Autodesk Fusion 360 part; units mm, degrees
(part 2 of 2)
sketch "Sketch2 (3)" plane through (0, 0, -6.4) normal (0, 0, -1) x (1, 0, 0) in component "Holding Plate"
  arc A0 (121.6882, 36.141) -> (112.1882, 45.641) centre (112.1882, 36.141) ccw
  line L0 (112.1882, 45.641) -> (14.8614, 45.641)
  line L1 (14.8614, 45.641) -> (14.8614, -58.688)
  line L2 (14.8614, -58.688) -> (98.2844, -58.688)
  line L3 (98.2844, -58.688) -> (98.2844, -66.2117)
  line L4 (98.2844, -66.2117) -> (121.1297, -66.2117)
  line L5 (121.1297, -66.2117) -> (121.1297, -42.1871)
  line L6 (121.1297, -42.1871) -> (101.4385, -42.1871)
  line L7 (101.4385, -42.1871) -> (101.4385, 27.1211)
  line L8 (101.4385, 27.1211) -> (121.6882, 27.1211)
  line L9 (121.6882, 27.1211) -> (121.6882, 36.141)
  line L10 (20, -40) -> (27.5, -40)
  line L11 (27.5, -40) -> (27.5, -43)
  line L12 (27.5, -43) -> (30.5, -43)
  line L13 (30.5, -43) -> (30.5, -49.2)
  line L14 (30.5, -49.2) -> (25.4, -49.2)
  line L15 (25.4, -49.2) -> (25.4, -54.4)
  line L16 (25.4, -54.4) -> (20, -54.4)
  line L17 (20, -54.4) -> (20, -40)
  line L18 (73.4, -1.6) -> (73.4, 0)
  line L19 (73.4, 0) -> (75, 0)
  line L20 (75, 0) -> (75, -1.6)
  line L21 (75, -1.6) -> (73.4, -1.6)
  line L22 (60, -40) -> (67.5, -40)
  line L23 (67.5, -40) -> (67.5, -43)
  line L24 (67.5, -43) -> (70.5, -43)
  line L25 (70.5, -43) -> (70.5, -49.2)
  line L26 (70.5, -49.2) -> (65.4, -49.2)
  line L27 (65.4, -49.2) -> (65.4, -54.4)
  line L28 (65.4, -54.4) -> (60, -54.4)
  line L29 (60, -54.4) -> (60, -40)
  line L30 (33.4, -41.6) -> (33.4, -40)
  line L31 (33.4, -40) -> (35, -40)
  line L32 (35, -40) -> (35, -41.6)
  line L33 (35, -41.6) -> (33.4, -41.6)
  line L34 (80, 20) -> (87.5, 20)
  line L35 (87.5, 20) -> (87.5, 17)
  line L36 (87.5, 17) -> (90.5, 17)
  line L37 (90.5, 17) -> (90.5, 10.8)
  line L38 (90.5, 10.8) -> (85.4, 10.8)
  line L39 (85.4, 10.8) -> (85.4, 5.6)
  line L40 (85.4, 5.6) -> (80, 5.6)
  line L41 (80, 5.6) -> (80, 20)
  line L42 (53.4, -41.6) -> (53.4, -40)
  line L43 (53.4, -40) -> (55, -40)
  line L44 (55, -40) -> (55, -41.6)
  line L45 (55, -41.6) -> (53.4, -41.6)
  line L46 (93.4, -1.6) -> (93.4, 0)
  line L47 (93.4, 0) -> (95, 0)
  line L48 (95, 0) -> (95, -1.6)
  line L49 (95, -1.6) -> (93.4, -1.6)
  line L50 (75, -52.8) -> (75, -54.4)
  line L51 (75, -54.4) -> (73.4, -54.4)
  line L52 (73.4, -54.4) -> (73.4, -52.8)
  line L53 (73.4, -52.8) -> (75, -52.8)
  line L54 (40, -40) -> (47.5, -40)
  line L55 (47.5, -40) -> (47.5, -43)
  line L56 (47.5, -43) -> (50.5, -43)
  line L57 (50.5, -43) -> (50.5, -49.2)
  line L58 (50.5, -49.2) -> (45.4, -49.2)
  line L59 (45.4, -49.2) -> (45.4, -54.4)
  line L60 (45.4, -54.4) -> (40, -54.4)
  line L61 (40, -54.4) -> (40, -40)
  line L62 (55, -52.8) -> (55, -54.4)
  line L63 (55, -54.4) -> (53.4, -54.4)
  line L64 (53.4, -54.4) -> (53.4, -52.8)
  line L65 (53.4, -52.8) -> (55, -52.8)
  line L66 (80, -20) -> (87.5, -20)
  line L67 (87.5, -20) -> (87.5, -23)
  line L68 (87.5, -23) -> (90.5, -23)
  line L69 (90.5, -23) -> (90.5, -29.2)
  line L70 (90.5, -29.2) -> (85.4, -29.2)
  line L71 (85.4, -29.2) -> (85.4, -34.4)
  line L72 (85.4, -34.4) -> (80, -34.4)
  line L73 (80, -34.4) -> (80, -20)
  line L74 (60, -20) -> (67.5, -20)
  line L75 (67.5, -20) -> (67.5, -23)
  line L76 (67.5, -23) -> (70.5, -23)
  line L77 (70.5, -23) -> (70.5, -29.2)
  line L78 (70.5, -29.2) -> (65.4, -29.2)
  line L79 (65.4, -29.2) -> (65.4, -34.4)
  line L80 (65.4, -34.4) -> (60, -34.4)
  line L81 (60, -34.4) -> (60, -20)
  line L82 (93.4, -21.6) -> (93.4, -20)
  line L83 (93.4, -20) -> (95, -20)
  line L84 (95, -20) -> (95, -21.6)
  line L85 (95, -21.6) -> (93.4, -21.6)
  line L86 (80, -40) -> (87.5, -40)
  line L87 (87.5, -40) -> (87.5, -43)
  line L88 (87.5, -43) -> (90.5, -43)
  line L89 (90.5, -43) -> (90.5, -49.2)
  line L90 (90.5, -49.2) -> (85.4, -49.2)
  line L91 (85.4, -49.2) -> (85.4, -54.4)
  line L92 (85.4, -54.4) -> (80, -54.4)
  line L93 (80, -54.4) -> (80, -40)
  line L94 (95, -54.4) -> (93.4, -54.4)
  line L95 (93.4, -54.4) -> (93.4, -52.8)
  line L96 (93.4, -52.8) -> (95, -52.8)
  line L97 (95, -52.8) -> (95, -54.4)
  line L98 (35, -52.8) -> (35, -54.4)
  line L99 (35, -54.4) -> (33.4, -54.4)
  line L100 (33.4, -54.4) -> (33.4, -52.8)
  line L101 (33.4, -52.8) -> (35, -52.8)
  line L102 (95, -12.8) -> (95, -14.4)
  line L103 (95, -14.4) -> (93.4, -14.4)
  line L104 (93.4, -14.4) -> (93.4, -12.8)
  line L105 (93.4, -12.8) -> (95, -12.8)
  line L106 (60, 0) -> (67.5, 0)
  line L107 (67.5, 0) -> (67.5, -3)
  line L108 (67.5, -3) -> (70.5, -3)
  line L109 (70.5, -3) -> (70.5, -9.2)
  line L110 (70.5, -9.2) -> (65.4, -9.2)
  line L111 (65.4, -9.2) -> (65.4, -14.4)
  line L112 (65.4, -14.4) -> (60, -14.4)
  line L113 (60, -14.4) -> (60, 0)
  line L114 (75, 7.2) -> (75, 5.6)
  line L115 (75, 5.6) -> (73.4, 5.6)
  line L116 (73.4, 5.6) -> (73.4, 7.2)
  line L117 (73.4, 7.2) -> (75, 7.2)
  line L118 (73.4, -21.6) -> (73.4, -20)
  line L119 (73.4, -20) -> (75, -20)
  line L120 (75, -20) -> (75, -21.6)
  line L121 (75, -21.6) -> (73.4, -21.6)
  line L122 (73.4, -41.6) -> (73.4, -40)
  line L123 (73.4, -40) -> (75, -40)
  line L124 (75, -40) -> (75, -41.6)
  line L125 (75, -41.6) -> (73.4, -41.6)
  line L126 (95, -32.8) -> (95, -34.4)
  line L127 (95, -34.4) -> (93.4, -34.4)
  line L128 (93.4, -34.4) -> (93.4, -32.8)
  line L129 (93.4, -32.8) -> (95, -32.8)
  line L130 (75, -32.8) -> (75, -34.4)
  line L131 (75, -34.4) -> (73.4, -34.4)
  line L132 (73.4, -34.4) -> (73.4, -32.8)
  line L133 (73.4, -32.8) -> (75, -32.8)
  line L134 (93.4, 18.4) -> (93.4, 20)
  line L135 (93.4, 20) -> (95, 20)
  line L136 (95, 20) -> (95, 18.4)
  line L137 (95, 18.4) -> (93.4, 18.4)
  line L138 (95, 7.2) -> (95, 5.6)
  line L139 (95, 5.6) -> (93.4, 5.6)
  line L140 (93.4, 5.6) -> (93.4, 7.2)
  line L141 (93.4, 7.2) -> (95, 7.2)
  line L142 (93.4, -41.6) -> (93.4, -40)
  line L143 (93.4, -40) -> (95, -40)
  line L144 (95, -40) -> (95, -41.6)
  line L145 (95, -41.6) -> (93.4, -41.6)
  line L146 (75, -12.8) -> (75, -14.4)
  line L147 (75, -14.4) -> (73.4, -14.4)
  line L148 (73.4, -14.4) -> (73.4, -12.8)
  line L149 (73.4, -12.8) -> (75, -12.8)
  line L150 (80, 0) -> (87.5, 0)
  line L151 (87.5, 0) -> (87.5, -3)
  line L152 (87.5, -3) -> (90.5, -3)
  line L153 (90.5, -3) -> (90.5, -9.2)
  line L154 (90.5, -9.2) -> (85.4, -9.2)
  line L155 (85.4, -9.2) -> (85.4, -14.4)
  line L156 (85.4, -14.4) -> (80, -14.4)
  line L157 (80, -14.4) -> (80, 0)
  line L158 (73.4, 18.4) -> (73.4, 20)
  line L159 (73.4, 20) -> (75, 20)
  line L160 (75, 20) -> (75, 18.4)
  line L161 (75, 18.4) -> (73.4, 18.4)
  line L162 (60, 20) -> (67.5, 20)
  line L163 (67.5, 20) -> (67.5, 17)
  line L164 (67.5, 17) -> (70.5, 17)
  line L165 (70.5, 17) -> (70.5, 10.8)
  line L166 (70.5, 10.8) -> (65.4, 10.8)
  line L167 (65.4, 10.8) -> (65.4, 5.6)
  line L168 (65.4, 5.6) -> (60, 5.6)
  line L169 (60, 5.6) -> (60, 20)
  line L170 (40, 40) -> (47.5, 40)
  line L171 (47.5, 40) -> (47.5, 37)
  line L172 (47.5, 37) -> (50.5, 37)
  line L173 (50.5, 37) -> (50.5, 30.8)
  line L174 (50.5, 30.8) -> (45.4, 30.8)
  line L175 (45.4, 30.8) -> (45.4, 25.6)
  line L176 (45.4, 25.6) -> (40, 25.6)
  line L177 (40, 25.6) -> (40, 40)
  line L178 (55, 27.2) -> (55, 25.6)
  line L179 (55, 25.6) -> (53.4, 25.6)
  line L180 (53.4, 25.6) -> (53.4, 27.2)
  line L181 (53.4, 27.2) -> (55, 27.2)
  line L182 (60, 40) -> (67.5, 40)
  line L183 (67.5, 40) -> (67.5, 37)
  line L184 (67.5, 37) -> (70.5, 37)
  line L185 (70.5, 37) -> (70.5, 30.8)
  line L186 (70.5, 30.8) -> (65.4, 30.8)
  line L187 (65.4, 30.8) -> (65.4, 25.6)
  line L188 (65.4, 25.6) -> (60, 25.6)
  line L189 (60, 25.6) -> (60, 40)
  line L190 (80, 40) -> (87.5, 40)
  line L191 (87.5, 40) -> (87.5, 37)
  line L192 (87.5, 37) -> (90.5, 37)
  line L193 (90.5, 37) -> (90.5, 30.8)
  line L194 (90.5, 30.8) -> (85.4, 30.8)
  line L195 (85.4, 30.8) -> (85.4, 25.6)
  line L196 (85.4, 25.6) -> (80, 25.6)
  line L197 (80, 25.6) -> (80, 40)
  line L198 (93.4, 38.4) -> (93.4, 40)
  line L199 (93.4, 40) -> (95, 40)
  line L200 (95, 40) -> (95, 38.4)
  line L201 (95, 38.4) -> (93.4, 38.4)
  line L202 (95, 27.2) -> (95, 25.6)
  line L203 (95, 25.6) -> (93.4, 25.6)
  line L204 (93.4, 25.6) -> (93.4, 27.2)
  line L205 (93.4, 27.2) -> (95, 27.2)
  line L206 (53.4, 38.4) -> (53.4, 40)
  line L207 (53.4, 40) -> (55, 40)
  line L208 (55, 40) -> (55, 38.4)
  line L209 (55, 38.4) -> (53.4, 38.4)
  line L210 (75, 27.2) -> (75, 25.6)
  line L211 (75, 25.6) -> (73.4, 25.6)
  line L212 (73.4, 25.6) -> (73.4, 27.2)
  line L213 (73.4, 27.2) -> (75, 27.2)
  line L214 (73.4, 38.4) -> (73.4, 40)
  line L215 (73.4, 40) -> (75, 40)
  line L216 (75, 40) -> (75, 38.4)
  line L217 (75, 38.4) -> (73.4, 38.4)
  circle A1 centre (28.0569, 26.8711) radius 5
  circle A2 centre (36.7164, -15.9226) radius 5
  circle A3 centre (109.0489, 35.4607) radius 5
  circle A4 centre (109.0489, -55.2728) radius 5
  dimension "d163" = 10
  dimension "d164" = 10
  dimension "d189" = 10
  dimension "d190" = 10
  measures "d163" diameter of A1
  measures "d164" diameter of A2
  measures "d189" diameter of A3
  measures "d190" diameter of A4
extrude "Extrude2''" add sketch "Sketch2 (3)" along normal blind 14.5 contours A1 | A2 | A3 | A4 bodies 3 in component "Holding Plate"
sketch "Sketch3 (3)" plane through (0, 0, 0) normal (0, 0, -1) x (1, 0, 0)
  arc A0 (123.05, 36.8) -> (113.05, 46.8) centre (113.05, 36.8) ccw
  line L0 (113.05, 46.8) -> (-34, 46.8)
  arc A1 (-34, 46.8) -> (-44, 36.8) centre (-34, 36.8) ccw
  line L1 (-44, 36.8) -> (-44, -87.5)
  arc A2 (-44, -87.5) -> (-34, -97.5) centre (-34, -87.5) ccw
  line L2 (-34, -97.5) -> (27.575, -97.5)
  line L3 (27.575, -97.5) -> (27.575, -75.5)
  line L4 (27.575, -75.5) -> (30.425, -75.5)
  line L5 (30.425, -75.5) -> (30.425, -97.5)
  line L6 (48.625, -97.5) -> (48.625, -75.5)
  line L7 (48.625, -75.5) -> (51.475, -75.5)
  line L8 (51.475, -75.5) -> (51.475, -97.5)
  line L9 (51.475, -97.5) -> (113.05, -97.5)
  arc A3 (113.05, -97.5) -> (123.05, -87.5) centre (113.05, -87.5) ccw
  line L10 (123.05, -87.5) -> (123.05, 36.8)
  line L11 (59.4, -55.25) -> (59.4, -39.15)
  line L12 (59.4, -39.15) -> (75.6, -39.15)
  line L13 (75.6, -39.15) -> (75.6, -55.25)
  line L14 (75.6, -55.25) -> (59.4, -55.25)
  line L15 (59.4, -15.25) -> (59.4, 0.85)
  line L16 (59.4, 0.85) -> (75.6, 0.85)
  line L17 (75.6, 0.85) -> (75.6, -15.25)
  line L18 (75.6, -15.25) -> (59.4, -15.25)
  line L19 (39.4, 24.75) -> (39.4, 40.85)
  line L20 (39.4, 40.85) -> (55.6, 40.85)
  line L21 (55.6, 40.85) -> (55.6, 24.75)
  line L22 (55.6, 24.75) -> (39.4, 24.75)
  line L23 (59.4, 24.75) -> (59.4, 40.85)
  line L24 (59.4, 40.85) -> (75.6, 40.85)
  line L25 (75.6, 40.85) -> (75.6, 24.75)
  line L26 (75.6, 24.75) -> (59.4, 24.75)
  line L27 (79.4, -15.25) -> (79.4, 0.85)
  line L28 (79.4, 0.85) -> (95.6, 0.85)
  line L29 (95.6, 0.85) -> (95.6, -15.25)
  line L30 (95.6, -15.25) -> (79.4, -15.25)
  line L31 (79.4, -55.25) -> (79.4, -39.15)
  line L32 (79.4, -39.15) -> (95.6, -39.15)
  line L33 (95.6, -39.15) -> (95.6, -55.25)
  line L34 (95.6, -55.25) -> (79.4, -55.25)
  line L35 (39.4, -55.25) -> (39.4, -39.15)
  line L36 (39.4, -39.15) -> (55.6, -39.15)
  line L37 (55.6, -39.15) -> (55.6, -55.25)
  line L38 (55.6, -55.25) -> (39.4, -55.25)
  line L39 (79.4, -35.25) -> (79.4, -19.15)
  line L40 (79.4, -19.15) -> (95.6, -19.15)
  line L41 (95.6, -19.15) -> (95.6, -35.25)
  line L42 (95.6, -35.25) -> (79.4, -35.25)
  line L43 (59.4, 4.75) -> (59.4, 20.85)
  line L44 (59.4, 20.85) -> (75.6, 20.85)
  line L45 (75.6, 20.85) -> (75.6, 4.75)
  line L46 (75.6, 4.75) -> (59.4, 4.75)
  line L47 (79.4, 24.75) -> (79.4, 40.85)
  line L48 (79.4, 40.85) -> (95.6, 40.85)
  line L49 (95.6, 40.85) -> (95.6, 24.75)
  line L50 (95.6, 24.75) -> (79.4, 24.75)
  line L51 (79.4, 4.75) -> (79.4, 20.85)
  line L52 (79.4, 20.85) -> (95.6, 20.85)
  line L53 (95.6, 20.85) -> (95.6, 4.75)
  line L54 (95.6, 4.75) -> (79.4, 4.75)
  line L55 (59.4, -35.25) -> (59.4, -19.15)
  line L56 (59.4, -19.15) -> (75.6, -19.15)
  line L57 (75.6, -19.15) -> (75.6, -35.25)
  line L58 (75.6, -35.25) -> (59.4, -35.25)
  line L59 (19.4, -55.25) -> (19.4, -39.15)
  line L60 (19.4, -39.15) -> (35.6, -39.15)
  line L61 (35.6, -39.15) -> (35.6, -55.25)
  line L62 (35.6, -55.25) -> (19.4, -55.25)
  circle A4 centre (112, -33.75) radius 2.75
  circle A5 centre (112, 19.35) radius 2.75
  circle A6 centre (-20.7, -75) radius 3.675
  circle A7 centre (19.3, -75) radius 3.675
  circle A8 centre (59.3, -75) radius 3.675
  circle A9 centre (99.3, -75) radius 3.675
  circle A10 centre (112, -7.2) radius 6.25
  circle A11 centre (0, 0) radius 3.675
  circle A12 centre (-26.1553, -31.0832) radius 5
  circle A13 centre (80.0291, -77.7504) radius 5
  circle A14 centre (-20.8711, 13.9931) radius 5
  line L63 (30.425, -97.5) -> (48.625, -97.5)
  circle A15 centre (-1.1738, -82.7474) radius 5
  dimension "d167" = 10
  dimension "d170" = 10
  dimension "d171" = 10
  dimension "d176" = 10
  measures "d167" diameter of A12
  measures "d170" diameter of A13
  measures "d171" diameter of A14
  measures "d176" diameter of A15
extrude "Extrude14" add sketch "Sketch3 (3)" along normal blind 21 contours A12 | A13 | A14 | A15 bodies 1 in component "Top"
sketch "Sketch11" plane through (0, 0, 0) normal (0, 0, -1) x (1, 0, 0) in component "Top"
  circle A0 centre (-1.1738, -82.7474) radius 5
  circle A1 centre (-26.1553, -31.0832) radius 5
  circle A2 centre (80.0291, -77.7504) radius 5
  circle A3 centre (-20.8711, 13.9931) radius 5
  arc A4 (123.05, 36.8) -> (113.05, 46.8) centre (113.05, 36.8) ccw
  line L0 (113.05, 46.8) -> (-34, 46.8)
  arc A5 (-34, 46.8) -> (-44, 36.8) centre (-34, 36.8) ccw
  line L1 (-44, 36.8) -> (-44, -87.5)
  arc A6 (-44, -87.5) -> (-34, -97.5) centre (-34, -87.5) ccw
  line L2 (-34, -97.5) -> (27.575, -97.5)
  line L3 (27.575, -97.5) -> (27.575, -75.5)
  line L4 (27.575, -75.5) -> (30.425, -75.5)
  line L5 (30.425, -75.5) -> (30.425, -97.5)
  line L6 (30.425, -97.5) -> (48.625, -97.5)
  line L7 (48.625, -97.5) -> (48.625, -75.5)
  line L8 (48.625, -75.5) -> (51.475, -75.5)
  line L9 (51.475, -75.5) -> (51.475, -97.5)
  line L10 (51.475, -97.5) -> (113.05, -97.5)
  arc A7 (113.05, -97.5) -> (123.05, -87.5) centre (113.05, -87.5) ccw
  line L11 (123.05, -87.5) -> (123.05, 36.8)
  line L12 (59.4, -55.25) -> (59.4, -39.15)
  line L13 (59.4, -39.15) -> (75.6, -39.15)
  line L14 (75.6, -39.15) -> (75.6, -55.25)
  line L15 (75.6, -55.25) -> (59.4, -55.25)
  line L16 (59.4, -15.25) -> (59.4, 0.85)
  line L17 (59.4, 0.85) -> (75.6, 0.85)
  line L18 (75.6, 0.85) -> (75.6, -15.25)
  line L19 (75.6, -15.25) -> (59.4, -15.25)
  line L20 (39.4, 24.75) -> (39.4, 40.85)
  line L21 (39.4, 40.85) -> (55.6, 40.85)
  line L22 (55.6, 40.85) -> (55.6, 24.75)
  line L23 (55.6, 24.75) -> (39.4, 24.75)
  line L24 (59.4, 24.75) -> (59.4, 40.85)
  line L25 (59.4, 40.85) -> (75.6, 40.85)
  line L26 (75.6, 40.85) -> (75.6, 24.75)
  line L27 (75.6, 24.75) -> (59.4, 24.75)
  line L28 (79.4, -15.25) -> (79.4, 0.85)
  line L29 (79.4, 0.85) -> (95.6, 0.85)
  line L30 (95.6, 0.85) -> (95.6, -15.25)
  line L31 (95.6, -15.25) -> (79.4, -15.25)
  line L32 (79.4, -55.25) -> (79.4, -39.15)
  line L33 (79.4, -39.15) -> (95.6, -39.15)
  line L34 (95.6, -39.15) -> (95.6, -55.25)
  line L35 (95.6, -55.25) -> (79.4, -55.25)
  line L36 (39.4, -55.25) -> (39.4, -39.15)
  line L37 (39.4, -39.15) -> (55.6, -39.15)
  line L38 (55.6, -39.15) -> (55.6, -55.25)
  line L39 (55.6, -55.25) -> (39.4, -55.25)
  line L40 (79.4, -35.25) -> (79.4, -19.15)
  line L41 (79.4, -19.15) -> (95.6, -19.15)
  line L42 (95.6, -19.15) -> (95.6, -35.25)
  line L43 (95.6, -35.25) -> (79.4, -35.25)
  line L44 (59.4, 4.75) -> (59.4, 20.85)
  line L45 (59.4, 20.85) -> (75.6, 20.85)
  line L46 (75.6, 20.85) -> (75.6, 4.75)
  line L47 (75.6, 4.75) -> (59.4, 4.75)
  line L48 (79.4, 24.75) -> (79.4, 40.85)
  line L49 (79.4, 40.85) -> (95.6, 40.85)
  line L50 (95.6, 40.85) -> (95.6, 24.75)
  line L51 (95.6, 24.75) -> (79.4, 24.75)
  line L52 (79.4, 4.75) -> (79.4, 20.85)
  line L53 (79.4, 20.85) -> (95.6, 20.85)
  line L54 (95.6, 20.85) -> (95.6, 4.75)
  line L55 (95.6, 4.75) -> (79.4, 4.75)
  line L56 (59.4, -35.25) -> (59.4, -19.15)
  line L57 (59.4, -19.15) -> (75.6, -19.15)
  line L58 (75.6, -19.15) -> (75.6, -35.25)
  line L59 (75.6, -35.25) -> (59.4, -35.25)
  line L60 (19.4, -55.25) -> (19.4, -39.15)
  line L61 (19.4, -39.15) -> (35.6, -39.15)
  line L62 (35.6, -39.15) -> (35.6, -55.25)
  line L63 (35.6, -55.25) -> (19.4, -55.25)
  circle A8 centre (112, -33.75) radius 2.75
  circle A9 centre (112, 19.35) radius 2.75
  circle A10 centre (-20.7, -75) radius 3.675
  circle A11 centre (19.3, -75) radius 3.675
  circle A12 centre (59.3, -75) radius 3.675
  circle A13 centre (99.3, -75) radius 3.675
  circle A14 centre (112, -7.2) radius 6.25
  circle A15 centre (0, 0) radius 3.675
  circle A16 centre (35.815, -26.5694) radius 5
  circle A17 centre (34.6117, 12.124) radius 5
  circle A18 centre (109.9321, -52.4845) radius 5
  circle A19 centre (107.0903, 35.1385) radius 5
  dimension "d177" = 10
  dimension "d178" = 10
  dimension "d179" = 10
  dimension "d180" = 10
  measures "d177" diameter of A16
  measures "d178" diameter of A17
  measures "d179" diameter of A18
  measures "d180" diameter of A19
extrude "Extrude15" add sketch "Sketch11" along normal blind 5.2 contours A16 | A17 | A18 bodies 1 in component "Top"
sketch "Sketch3 (4)" plane through (0, 0, -4.4) normal (0, 0, 1) x (-1, 0, 0) in component "Holding Plate"
  arc A0 (-112.1882, 45.641) -> (-121.6882, 36.141) centre (-112.1882, 36.141) ccw
  line L0 (-121.6882, 36.141) -> (-121.6882, 27.1211)
  line L1 (-121.6882, 27.1211) -> (-101.4385, 27.1211)
  line L2 (-101.4385, 27.1211) -> (-101.4385, -42.1871)
  line L3 (-101.4385, -42.1871) -> (-121.1297, -42.1871)
  line L4 (-121.1297, -42.1871) -> (-121.1297, -66.2117)
  line L5 (-121.1297, -66.2117) -> (-98.2844, -66.2117)
  line L6 (-98.2844, -66.2117) -> (-98.2844, -58.688)
  line L7 (-98.2844, -58.688) -> (-14.8614, -58.688)
  line L8 (-14.8614, -58.688) -> (-14.8614, 45.641)
  line L9 (-14.8614, 45.641) -> (-112.1882, 45.641)
  line L10 (-93.4, -54.4) -> (-95, -54.4)
  line L11 (-95, -54.4) -> (-95, -52.8)
  line L12 (-95, -52.8) -> (-93.4, -52.8)
  line L13 (-93.4, -52.8) -> (-93.4, -54.4)
  line L14 (-93.4, -40) -> (-93.4, -41.6)
  line L15 (-93.4, -41.6) -> (-95, -41.6)
  line L16 (-95, -41.6) -> (-95, -40)
  line L17 (-95, -40) -> (-93.4, -40)
  line L18 (-73.4, -40) -> (-73.4, -41.6)
  line L19 (-73.4, -41.6) -> (-75, -41.6)
  line L20 (-75, -41.6) -> (-75, -40)
  line L21 (-75, -40) -> (-73.4, -40)
  line L22 (-87.5, -40) -> (-80, -40)
  line L23 (-80, -40) -> (-80, -54.4)
  line L24 (-80, -54.4) -> (-85.4, -54.4)
  line L25 (-85.4, -54.4) -> (-85.4, -49.2)
  line L26 (-85.4, -49.2) -> (-90.5, -49.2)
  line L27 (-90.5, -49.2) -> (-90.5, -43)
  line L28 (-90.5, -43) -> (-87.5, -43)
  line L29 (-87.5, -43) -> (-87.5, -40)
  line L30 (-75, -54.4) -> (-75, -52.8)
  line L31 (-75, -52.8) -> (-73.4, -52.8)
  line L32 (-73.4, -52.8) -> (-73.4, -54.4)
  line L33 (-73.4, -54.4) -> (-75, -54.4)
  line L34 (-47.5, -40) -> (-40, -40)
  line L35 (-40, -40) -> (-40, -54.4)
  line L36 (-40, -54.4) -> (-45.4, -54.4)
  line L37 (-45.4, -54.4) -> (-45.4, -49.2)
  line L38 (-45.4, -49.2) -> (-50.5, -49.2)
  line L39 (-50.5, -49.2) -> (-50.5, -43)
  line L40 (-50.5, -43) -> (-47.5, -43)
  line L41 (-47.5, -43) -> (-47.5, -40)
  line L42 (-87.5, 0) -> (-80, 0)
  line L43 (-80, 0) -> (-80, -14.4)
  line L44 (-80, -14.4) -> (-85.4, -14.4)
  line L45 (-85.4, -14.4) -> (-85.4, -9.2)
  line L46 (-85.4, -9.2) -> (-90.5, -9.2)
  line L47 (-90.5, -9.2) -> (-90.5, -3)
  line L48 (-90.5, -3) -> (-87.5, -3)
  line L49 (-87.5, -3) -> (-87.5, 0)
  line L50 (-87.5, -20) -> (-80, -20)
  line L51 (-80, -20) -> (-80, -34.4)
  line L52 (-80, -34.4) -> (-85.4, -34.4)
  line L53 (-85.4, -34.4) -> (-85.4, -29.2)
  line L54 (-85.4, -29.2) -> (-90.5, -29.2)
  line L55 (-90.5, -29.2) -> (-90.5, -23)
  line L56 (-90.5, -23) -> (-87.5, -23)
  line L57 (-87.5, -23) -> (-87.5, -20)
  line L58 (-75, -14.4) -> (-75, -12.8)
  line L59 (-75, -12.8) -> (-73.4, -12.8)
  line L60 (-73.4, -12.8) -> (-73.4, -14.4)
  line L61 (-73.4, -14.4) -> (-75, -14.4)
  line L62 (-73.4, 0) -> (-73.4, -1.6)
  line L63 (-73.4, -1.6) -> (-75, -1.6)
  line L64 (-75, -1.6) -> (-75, 0)
  line L65 (-75, 0) -> (-73.4, 0)
  line L66 (-95, -14.4) -> (-95, -12.8)
  line L67 (-95, -12.8) -> (-93.4, -12.8)
  line L68 (-93.4, -12.8) -> (-93.4, -14.4)
  line L69 (-93.4, -14.4) -> (-95, -14.4)
  line L70 (-95, -34.4) -> (-95, -32.8)
  line L71 (-95, -32.8) -> (-93.4, -32.8)
  line L72 (-93.4, -32.8) -> (-93.4, -34.4)
  line L73 (-93.4, -34.4) -> (-95, -34.4)
  line L74 (-67.5, -40) -> (-60, -40)
  line L75 (-60, -40) -> (-60, -54.4)
  line L76 (-60, -54.4) -> (-65.4, -54.4)
  line L77 (-65.4, -54.4) -> (-65.4, -49.2)
  line L78 (-65.4, -49.2) -> (-70.5, -49.2)
  line L79 (-70.5, -49.2) -> (-70.5, -43)
  line L80 (-70.5, -43) -> (-67.5, -43)
  line L81 (-67.5, -43) -> (-67.5, -40)
  line L82 (-95, 5.6) -> (-95, 7.2)
  line L83 (-95, 7.2) -> (-93.4, 7.2)
  line L84 (-93.4, 7.2) -> (-93.4, 5.6)
  line L85 (-93.4, 5.6) -> (-95, 5.6)
  line L86 (-93.4, 20) -> (-93.4, 18.4)
  line L87 (-93.4, 18.4) -> (-95, 18.4)
  line L88 (-95, 18.4) -> (-95, 20)
  line L89 (-95, 20) -> (-93.4, 20)
  line L90 (-67.5, 0) -> (-60, 0)
  line L91 (-60, 0) -> (-60, -14.4)
  line L92 (-60, -14.4) -> (-65.4, -14.4)
  line L93 (-65.4, -14.4) -> (-65.4, -9.2)
  line L94 (-65.4, -9.2) -> (-70.5, -9.2)
  line L95 (-70.5, -9.2) -> (-70.5, -3)
  line L96 (-70.5, -3) -> (-67.5, -3)
  line L97 (-67.5, -3) -> (-67.5, 0)
  line L98 (-27.5, -40) -> (-20, -40)
  line L99 (-20, -40) -> (-20, -54.4)
  line L100 (-20, -54.4) -> (-25.4, -54.4)
  line L101 (-25.4, -54.4) -> (-25.4, -49.2)
  line L102 (-25.4, -49.2) -> (-30.5, -49.2)
  line L103 (-30.5, -49.2) -> (-30.5, -43)
  line L104 (-30.5, -43) -> (-27.5, -43)
  line L105 (-27.5, -43) -> (-27.5, -40)
  line L106 (-73.4, -20) -> (-73.4, -21.6)
  line L107 (-73.4, -21.6) -> (-75, -21.6)
  line L108 (-75, -21.6) -> (-75, -20)
  line L109 (-75, -20) -> (-73.4, -20)
  line L110 (-67.5, -20) -> (-60, -20)
  line L111 (-60, -20) -> (-60, -34.4)
  line L112 (-60, -34.4) -> (-65.4, -34.4)
  line L113 (-65.4, -34.4) -> (-65.4, -29.2)
  line L114 (-65.4, -29.2) -> (-70.5, -29.2)
  line L115 (-70.5, -29.2) -> (-70.5, -23)
  line L116 (-70.5, -23) -> (-67.5, -23)
  line L117 (-67.5, -23) -> (-67.5, -20)
  line L118 (-75, -34.4) -> (-75, -32.8)
  line L119 (-75, -32.8) -> (-73.4, -32.8)
  line L120 (-73.4, -32.8) -> (-73.4, -34.4)
  line L121 (-73.4, -34.4) -> (-75, -34.4)
  line L122 (-33.4, -40) -> (-33.4, -41.6)
  line L123 (-33.4, -41.6) -> (-35, -41.6)
  line L124 (-35, -41.6) -> (-35, -40)
  line L125 (-35, -40) -> (-33.4, -40)
  line L126 (-93.4, 0) -> (-93.4, -1.6)
  line L127 (-93.4, -1.6) -> (-95, -1.6)
  line L128 (-95, -1.6) -> (-95, 0)
  line L129 (-95, 0) -> (-93.4, 0)
  line L130 (-55, -54.4) -> (-55, -52.8)
  line L131 (-55, -52.8) -> (-53.4, -52.8)
  line L132 (-53.4, -52.8) -> (-53.4, -54.4)
  line L133 (-53.4, -54.4) -> (-55, -54.4)
  line L134 (-93.4, -20) -> (-93.4, -21.6)
  line L135 (-93.4, -21.6) -> (-95, -21.6)
  line L136 (-95, -21.6) -> (-95, -20)
  line L137 (-95, -20) -> (-93.4, -20)
  line L138 (-35, -54.4) -> (-35, -52.8)
  line L139 (-35, -52.8) -> (-33.4, -52.8)
  line L140 (-33.4, -52.8) -> (-33.4, -54.4)
  line L141 (-33.4, -54.4) -> (-35, -54.4)
  line L142 (-53.4, -40) -> (-53.4, -41.6)
  line L143 (-53.4, -41.6) -> (-55, -41.6)
  line L144 (-55, -41.6) -> (-55, -40)
  line L145 (-55, -40) -> (-53.4, -40)
  line L146 (-75, 25.6) -> (-75, 27.2)
  line L147 (-75, 27.2) -> (-73.4, 27.2)
  line L148 (-73.4, 27.2) -> (-73.4, 25.6)
  line L149 (-73.4, 25.6) -> (-75, 25.6)
  line L150 (-93.4, 40) -> (-93.4, 38.4)
  line L151 (-93.4, 38.4) -> (-95, 38.4)
  line L152 (-95, 38.4) -> (-95, 40)
  line L153 (-95, 40) -> (-93.4, 40)
  line L154 (-73.4, 20) -> (-73.4, 18.4)
  line L155 (-73.4, 18.4) -> (-75, 18.4)
  line L156 (-75, 18.4) -> (-75, 20)
  line L157 (-75, 20) -> (-73.4, 20)
  line L158 (-75, 5.6) -> (-75, 7.2)
  line L159 (-75, 7.2) -> (-73.4, 7.2)
  line L160 (-73.4, 7.2) -> (-73.4, 5.6)
  line L161 (-73.4, 5.6) -> (-75, 5.6)
  line L162 (-53.4, 40) -> (-53.4, 38.4)
  line L163 (-53.4, 38.4) -> (-55, 38.4)
  line L164 (-55, 38.4) -> (-55, 40)
  line L165 (-55, 40) -> (-53.4, 40)
  line L166 (-55, 25.6) -> (-55, 27.2)
  line L167 (-55, 27.2) -> (-53.4, 27.2)
  line L168 (-53.4, 27.2) -> (-53.4, 25.6)
  line L169 (-53.4, 25.6) -> (-55, 25.6)
  line L170 (-95, 25.6) -> (-95, 27.2)
  line L171 (-95, 27.2) -> (-93.4, 27.2)
  line L172 (-93.4, 27.2) -> (-93.4, 25.6)
  line L173 (-93.4, 25.6) -> (-95, 25.6)
  line L174 (-87.5, 40) -> (-80, 40)
  line L175 (-80, 40) -> (-80, 25.6)
  line L176 (-80, 25.6) -> (-85.4, 25.6)
  line L177 (-85.4, 25.6) -> (-85.4, 30.8)
  line L178 (-85.4, 30.8) -> (-90.5, 30.8)
  line L179 (-90.5, 30.8) -> (-90.5, 37)
  line L180 (-90.5, 37) -> (-87.5, 37)
  line L181 (-87.5, 37) -> (-87.5, 40)
  line L182 (-87.5, 20) -> (-80, 20)
  line L183 (-80, 20) -> (-80, 5.6)
  line L184 (-80, 5.6) -> (-85.4, 5.6)
  line L185 (-85.4, 5.6) -> (-85.4, 10.8)
  line L186 (-85.4, 10.8) -> (-90.5, 10.8)
  line L187 (-90.5, 10.8) -> (-90.5, 17)
  line L188 (-90.5, 17) -> (-87.5, 17)
  line L189 (-87.5, 17) -> (-87.5, 20)
  line L190 (-73.4, 40) -> (-73.4, 38.4)
  line L191 (-73.4, 38.4) -> (-75, 38.4)
  line L192 (-75, 38.4) -> (-75, 40)
  line L193 (-75, 40) -> (-73.4, 40)
  line L194 (-47.5, 40) -> (-40, 40)
  line L195 (-40, 40) -> (-40, 25.6)
  line L196 (-40, 25.6) -> (-45.4, 25.6)
  line L197 (-45.4, 25.6) -> (-45.4, 30.8)
  line L198 (-45.4, 30.8) -> (-50.5, 30.8)
  line L199 (-50.5, 30.8) -> (-50.5, 37)
  line L200 (-50.5, 37) -> (-47.5, 37)
  line L201 (-47.5, 37) -> (-47.5, 40)
  line L202 (-67.5, 20) -> (-60, 20)
  line L203 (-60, 20) -> (-60, 5.6)
  line L204 (-60, 5.6) -> (-65.4, 5.6)
  line L205 (-65.4, 5.6) -> (-65.4, 10.8)
  line L206 (-65.4, 10.8) -> (-70.5, 10.8)
  line L207 (-70.5, 10.8) -> (-70.5, 17)
  line L208 (-70.5, 17) -> (-67.5, 17)
  line L209 (-67.5, 17) -> (-67.5, 20)
  line L210 (-67.5, 40) -> (-60, 40)
  line L211 (-60, 40) -> (-60, 25.6)
  line L212 (-60, 25.6) -> (-65.4, 25.6)
  line L213 (-65.4, 25.6) -> (-65.4, 30.8)
  line L214 (-65.4, 30.8) -> (-70.5, 30.8)
  line L215 (-70.5, 30.8) -> (-70.5, 37)
  line L216 (-70.5, 37) -> (-67.5, 37)
  line L217 (-67.5, 37) -> (-67.5, 40)
  circle A1 centre (-35.815, -26.5694) radius 5
  circle A2 centre (-34.6117, 12.124) radius 5
  circle A3 centre (-107.0903, 35.1385) radius 5
  circle A4 centre (-109.9321, -52.4845) radius 5
  circle A5 centre (-35.815, -26.5694) radius 5.2
  circle A6 centre (-34.6117, 12.124) radius 5.2
  circle A7 centre (-107.0903, 35.1385) radius 5.2
  circle A8 centre (-109.9321, -52.4845) radius 5.2
  dimension "d183" = 0.2
  dimension "d184" = 0.2
  dimension "d185" = 0.2
  dimension "d186" = 0.2
extrude "Extrude3'" cut sketch "Sketch3 (4)" against normal blind 1 contours A1 | A2 | A4 | A5 | A6 | A8 bodies 3 in component "Holding Plate"
sketch "Sketch2 (4)" plane through (0, 0, -24) normal (0, 0, -1) x (1, 0, 0) in component "Base"
  arc A0 (122.85, 36.8) -> (113.05, 46.6) centre (113.05, 36.8) ccw
  line L0 (113.05, 46.6) -> (-34, 46.6)
  arc A1 (-34, 46.6) -> (-43.8, 36.8) centre (-34, 36.8) ccw
  line L1 (-43.8, 36.8) -> (-43.8, -87.5)
  arc A2 (-43.8, -87.5) -> (-34, -97.3) centre (-34, -87.5) ccw
  line L2 (-34, -97.3) -> (113.05, -97.3)
  arc A3 (113.05, -97.3) -> (122.85, -87.5) centre (113.05, -87.5) ccw
  line L3 (122.85, -87.5) -> (122.85, 36.8)
  circle A4 centre (-20.8711, 13.9931) radius 5
  circle A5 centre (-26.1553, -31.0832) radius 5
  circle A6 centre (-1.1738, -82.7474) radius 5
  circle A7 centre (36.7164, -15.9226) radius 5
  circle A8 centre (28.0569, 26.8711) radius 5
  circle A9 centre (109.0489, -55.2728) radius 5
  circle A10 centre (80.0291, -77.7504) radius 5
  circle A11 centre (109.0489, 35.4607) radius 5
  circle A12 centre (36.7164, -15.9226) radius 1.3
  circle A13 centre (28.0569, 26.8711) radius 1.3
  circle A14 centre (-20.8711, 13.9931) radius 1.3
  circle A15 centre (-26.1553, -31.0832) radius 1.3
  circle A16 centre (-1.1738, -82.7474) radius 1.3
  circle A17 centre (80.0291, -77.7504) radius 1.3
  circle A18 centre (109.0489, -55.2728) radius 1.3
  circle A19 centre (109.0489, 35.4607) radius 1.3
  dimension "d192" = 2.6
  dimension "d193" = 2.6
  dimension "d194" = 2.6
  dimension "d195" = 2.6
  dimension "d196" = 2.6
  dimension "d197" = 2.6
  dimension "d198" = 2.6
  dimension "d199" = 2.6
  constraint concentric A7 A12
  constraint concentric A8 A13
  constraint concentric A4 A14
  constraint concentric A5 A15
  constraint concentric A6 A16
  constraint concentric A10 A17
  constraint concentric A9 A18
  constraint concentric A11 A19
  measures "d192" diameter of A12
  measures "d193" diameter of A13
  measures "d194" diameter of A14
  measures "d195" diameter of A15
  measures "d196" diameter of A16
  measures "d197" diameter of A17
  measures "d198" diameter of A18
  measures "d199" diameter of A19
extrude "Extrude16" cut sketch "Sketch2 (4)" against normal blind 15 contours A12 | A13 | A14 | A15 | A16 | A17 | A18 | A19 bodies 1 in component "Top"
extrude "Extrude4" cut sketch "Sketch2 (4)" against normal blind 15 contours A12 | A13 | A14 | A15 | A16 | A17 | A18 | A19 bodies 3 in component "Holding Plate"
extrude "Extrude2'''" cut sketch "Sketch2 (4)" against normal blind 15 contours A12 | A13 | A14 | A15 | A16 | A17 | A18 | A19 bodies 5 in component "Base"
chamfer "Chamfer1'" distance 2.75 angle 45 8 edges at (-27.3673, 30.6131, -24) (-2.3858, 82.2773, -24) (35.5044, 15.4525, -24) (26.8449, -27.3412, -24) (-22.0831, -14.4632, -24) (107.8369, -35.9308, -24) (107.8369, 54.8027, -24) (78.817, 77.2803, -24) on bodies 5 in component "Base"
fillet "Fillet6" radius 5 4 edges at (-30.8169, 29.2751, 0) (-25.5328, -15.8011, 0) (-5.8355, 80.9393, 0) (75.3674, 75.9423, 0) on bodies 1 in component "Top"
fillet "Fillet2'" radius 5 4 edges at (23.3952, -28.6792, -6.4) (32.0548, 14.1145, -6.4) (104.3873, -37.2687, -6.4) (104.3873, 53.4647, -6.4) on bodies 3 in component "Holding Plate"
sketch "Sketch12" plane through (0, 0, 0) normal (0, 0, -1) x (1, 0, 0) in component "Top"
  circle A0 centre (-1.1738, -82.7474) radius 10
  circle A1 centre (-26.1553, -31.0832) radius 10
  circle A2 centre (34.6117, 12.124) radius 5
  circle A3 centre (109.9321, -52.4845) radius 5
  circle A4 centre (35.815, -26.5694) radius 5
  arc A5 (123.05, 36.8) -> (113.05, 46.8) centre (113.05, 36.8) ccw
  line L0 (113.05, 46.8) -> (-34, 46.8)
  arc A6 (-34, 46.8) -> (-44, 36.8) centre (-34, 36.8) ccw
  line L1 (-44, 36.8) -> (-44, -87.5)
  arc A7 (-44, -87.5) -> (-34, -97.5) centre (-34, -87.5) ccw
  line L2 (-34, -97.5) -> (27.575, -97.5)
  line L3 (27.575, -97.5) -> (27.575, -75.5)
  line L4 (27.575, -75.5) -> (30.425, -75.5)
  line L5 (30.425, -75.5) -> (30.425, -97.5)
  line L6 (30.425, -97.5) -> (48.625, -97.5)
  line L7 (48.625, -97.5) -> (48.625, -75.5)
  line L8 (48.625, -75.5) -> (51.475, -75.5)
  line L9 (51.475, -75.5) -> (51.475, -97.5)
  line L10 (51.475, -97.5) -> (113.05, -97.5)
  arc A8 (113.05, -97.5) -> (123.05, -87.5) centre (113.05, -87.5) ccw
  line L11 (123.05, -87.5) -> (123.05, 36.8)
  line L12 (59.4, -55.25) -> (59.4, -39.15)
  line L13 (59.4, -39.15) -> (75.6, -39.15)
  line L14 (75.6, -39.15) -> (75.6, -55.25)
  line L15 (75.6, -55.25) -> (59.4, -55.25)
  line L16 (59.4, -15.25) -> (59.4, 0.85)
  line L17 (59.4, 0.85) -> (75.6, 0.85)
  line L18 (75.6, 0.85) -> (75.6, -15.25)
  line L19 (75.6, -15.25) -> (59.4, -15.25)
  line L20 (39.4, 24.75) -> (39.4, 40.85)
  line L21 (39.4, 40.85) -> (55.6, 40.85)
  line L22 (55.6, 40.85) -> (55.6, 24.75)
  line L23 (55.6, 24.75) -> (39.4, 24.75)
  line L24 (59.4, 24.75) -> (59.4, 40.85)
  line L25 (59.4, 40.85) -> (75.6, 40.85)
  line L26 (75.6, 40.85) -> (75.6, 24.75)
  line L27 (75.6, 24.75) -> (59.4, 24.75)
  line L28 (79.4, -15.25) -> (79.4, 0.85)
  line L29 (79.4, 0.85) -> (95.6, 0.85)
  line L30 (95.6, 0.85) -> (95.6, -15.25)
  line L31 (95.6, -15.25) -> (79.4, -15.25)
  line L32 (79.4, -55.25) -> (79.4, -39.15)
  line L33 (79.4, -39.15) -> (95.6, -39.15)
  line L34 (95.6, -39.15) -> (95.6, -55.25)
  line L35 (95.6, -55.25) -> (79.4, -55.25)
  line L36 (39.4, -55.25) -> (39.4, -39.15)
  line L37 (39.4, -39.15) -> (55.6, -39.15)
  line L38 (55.6, -39.15) -> (55.6, -55.25)
  line L39 (55.6, -55.25) -> (39.4, -55.25)
  line L40 (79.4, -35.25) -> (79.4, -19.15)
  line L41 (79.4, -19.15) -> (95.6, -19.15)
  line L42 (95.6, -19.15) -> (95.6, -35.25)
  line L43 (95.6, -35.25) -> (79.4, -35.25)
  line L44 (59.4, 4.75) -> (59.4, 20.85)
  line L45 (59.4, 20.85) -> (75.6, 20.85)
  line L46 (75.6, 20.85) -> (75.6, 4.75)
  line L47 (75.6, 4.75) -> (59.4, 4.75)
  line L48 (79.4, 24.75) -> (79.4, 40.85)
  line L49 (79.4, 40.85) -> (95.6, 40.85)
  line L50 (95.6, 40.85) -> (95.6, 24.75)
  line L51 (95.6, 24.75) -> (79.4, 24.75)
  line L52 (79.4, 4.75) -> (79.4, 20.85)
  line L53 (79.4, 20.85) -> (95.6, 20.85)
  line L54 (95.6, 20.85) -> (95.6, 4.75)
  line L55 (95.6, 4.75) -> (79.4, 4.75)
  line L56 (59.4, -35.25) -> (59.4, -19.15)
  line L57 (59.4, -19.15) -> (75.6, -19.15)
  line L58 (75.6, -19.15) -> (75.6, -35.25)
  line L59 (75.6, -35.25) -> (59.4, -35.25)
  line L60 (19.4, -55.25) -> (19.4, -39.15)
  line L61 (19.4, -39.15) -> (35.6, -39.15)
  line L62 (35.6, -39.15) -> (35.6, -55.25)
  line L63 (35.6, -55.25) -> (19.4, -55.25)
  circle A9 centre (-20.7, -75) radius 3.675
  circle A10 centre (112, 19.35) radius 2.75
  circle A11 centre (112, -33.75) radius 2.75
  circle A12 centre (19.3, -75) radius 3.675
  circle A13 centre (59.3, -75) radius 3.675
  circle A14 centre (99.3, -75) radius 3.675
  circle A15 centre (112, -7.2) radius 6.25
  circle A16 centre (0, 0) radius 3.675
  circle A17 centre (-20.8711, 13.9931) radius 10
  circle A18 centre (80.0291, -77.7504) radius 10
  circle A19 centre (109.0489, 35.4607) radius 5
  circle A20 centre (109.0489, 35.4607) radius 3.4
  circle A21 centre (109.0489, 35.4607) radius 3.8
  dimension "d211" = -1.6
  dimension "d212" = -1.2
extrude "Extrude5'" cut sketch "Sketch12" along normal blind 15.2 contours A20 | A21 bodies 3 in component "Holding Plate"
extrude "Extrude17" add sketch "Sketch12" along normal blind 15 contours A20 bodies 1 in component "Top"
sketch "Sketch13" plane through (0, 0, -15) normal (0, 0, -1) x (1, 0, 0) in component "Top"
  circle A0 centre (109.0489, 35.4607) radius 3.4
  circle A1 centre (109.0489, 35.4607) radius 1.3
  dimension "d217" = 2.6
  constraint concentric A0 A1
  measures "d217" diameter of A1
extrude "Extrude18" cut sketch "Sketch13" against normal blind 9 contours A1 bodies 1 in component "Top"
move_face "OffsetFaces1" offset -0.5 1 faces at (109.0813, -36.7602, -19) on bodies 3 in component "Holding Plate"
move_face "OffsetFaces1'" offset -0.5 8 faces at (109.0813, -36.7602, -21.1667) (109.0813, 53.9732, -21.1667) (81.1708, 77.1287, -21.1667) (36.7488, 14.623, -21.1667) (29.3504, -26.7417, -21.1667) (-2.2831, 83.4252, -21.0833) (-24.8617, 31.2126, -21.1667) (-21.9074, -14.778, -21.1667) on bodies 5 in component "Base"
fillet "Fillet7" radius 2.75 1 edges at (105.879, -36.6901, 0) on bodies 1 in component "Top"
sketch "Sketch3 (5)" plane through (0, 0, -24) normal (0, 0, -1) x (1, 0, 0) in component "Base"
  circle A0 centre (109.0489, -55.2728) radius 4.05
  circle A1 centre (-20.8711, 13.9931) radius 4.05
  circle A2 centre (36.7164, -15.9226) radius 4.05
  circle A3 centre (-26.1553, -31.0832) radius 4.05
  arc A4 (122.85, 36.8) -> (113.05, 46.6) centre (113.05, 36.8) ccw
  line L0 (113.05, 46.6) -> (-34, 46.6)
  arc A5 (-34, 46.6) -> (-43.8, 36.8) centre (-34, 36.8) ccw
  line L1 (-43.8, 36.8) -> (-43.8, -87.5)
  arc A6 (-43.8, -87.5) -> (-34, -97.3) centre (-34, -87.5) ccw
  line L2 (-34, -97.3) -> (113.05, -97.3)
  arc A7 (113.05, -97.3) -> (122.85, -87.5) centre (113.05, -87.5) ccw
  line L3 (122.85, -87.5) -> (122.85, 36.8)
  circle A8 centre (-1.1738, -82.7474) radius 4.05
  circle A9 centre (28.0569, 26.8711) radius 4.05
  circle A10 centre (109.0489, 35.4607) radius 4.05
  circle A11 centre (80.0291, -77.7504) radius 4.05
  line L4 (39.525, -97.3) -> (39.525, -93.3) construction
  line L5 (39.525, -93.3) -> (35.525, -93.3)
  line L6 (39.525, -93.3) -> (43.525, -93.3)
  line L7 (43.525, -93.3) -> (43.525, -97.3)
  line L8 (35.525, -93.3) -> (35.525, -97.3)
  line L9 (39.525, -97.3) -> (39.525, -68.8) construction
  circle A12 centre (39.525, -68.8) radius 3.5
  dimension "d225" = 4
  dimension "d226" = 4
  dimension "d227" = 4
  dimension "d231" = 28.5
  dimension "d232" = 7
  constraint midpoint L2 L4.start
  constraint perpendicular L2 L4
  constraint perpendicular L4 L5
  constraint perpendicular L4 L6
  constraint coincident L2 L7.end
  constraint perpendicular L2 L7
  constraint coincident L2 L8.end
  constraint perpendicular L2 L8
  constraint perpendicular L6 L9
  constraint coincident L9.end A12.centre
  measures "d225" distance of L4.start L4.end
  measures "d226" distance of L4.end L5.end
  measures "d227" distance of L4.end L6.end
  measures "d231" distance of L4.start L9.end
  measures "d232" diameter of A12
extrude "Extrude3''" cut sketch "Sketch3 (5)" against normal blind 3 contours L2 L5 L6 L7 L8 | A12 bodies 5 in component "Base"
sketch "Sketch4" plane through (0, 0, 3) normal (0, 0, -1) x (1, 0, 0) in component "Big Wheel"
  line L0 (-2.3331, 2.2193) -> (2.3613, 2.1893)
  arc A0 (-2.3331, 2.2193) -> (2.3613, 2.1893) centre (0, 0) ccw
  circle A1 centre (0, 0) radius 37
  circle A2 centre (0, 0) radius 10
  circle A3 centre (0, 0) radius 37
  dimension "d233" = 20
  constraint coincident A0.centre A1.centre
  measures "d233" diameter of A2
extrude "Extrude4'" add sketch "Sketch4" along normal blind 5 contours A1 A3 bodies 4 in component "Big Wheel"
component "Top" placed x (1, 0, 0) y (0, 1, 0) z (0, 0, 1) at (0, 0, 0)
component "Holding Plate" placed x (1, 0, 0) y (0, 1, 0) z (0, 0, 1) at (0, 0, 0)
component "Big Wheel" placed x (1, 0, 0) y (0, 1, 0) z (0, 0, 1) at (0, 0, 0)
component "Base" placed x (1, 0, 0) y (0, 1, 0) z (0, 0, 1) at (0, 0, 0)
equation "d8 = 13.75 mm + 0.65 mm"
equation "d101 = 180 deg - 60 deg"
equation "d165 = 11.50 mm + 3 mm"
